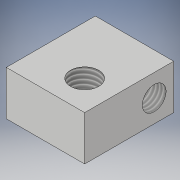
# Autodesk Inventor part: КВ33.000.109 - Каретка
Saved by Autodesk Inventor 2019 (Build 230136000, 136)
## iProperties
Created: 2021-04-04
Part Number: КВ33.000.109 - Каретка
Material: Типовые
Document SubType Name: Modeling
Designer: Петров Иван
Density: 1 g/cm^3
Appearance: По умолчанию
Mass: 10.7217 g
Surface Area: 35.9412 cm^2
Volume: 10.7217 cm^3
Author: Петров Иван
Autodesk Inventor part; units mm, degrees
ref_plane "YZ Plane" through (0, 0, 0) normal (1, 0, 0) x (0, 1, 0)
ref_plane "XZ Plane" through (0, 0, 0) normal (0, 1, 0) x (-1, 0, 0)
ref_plane "XY Plane" through (0, 0, 0) normal (0, 0, 1) x (1, 0, 0)
sketch "Sketch1" plane through (0, 0, 0) normal (0, 1, 0) x (-1, 0, 0)
  line L0 (0, 0) -> (26.4, 0)
  line L1 (26.4, 0) -> (26.4, -30)
  line L2 (26.4, -30) -> (0, -30)
  line L3 (0, -30) -> (0, 0)
  dimension "d0" = 26.4
  dimension "d1" = 30
  constraints: 8 end point, 2 parallel, 1 horizontal, 1 perpendicular
  measures "d0" distance of L1.end L2.end
  measures "d1" distance between parallel lines of L2 L0
extrude "Extrusion1" add sketch "Sketch1" along normal blind 15
sketch "Sketch2" plane through (0, 15, 0) normal (0, 1, 0) x (1, 0, 0)
  circle A0 centre (-10, 10) radius 4.75
  line L0 (0, 0) -> (0, 30) projected
  line L1 (-26.4, 0) -> (0, 0) projected
  dimension "d4" = 9.5
  dimension "d5" = 10
  dimension "d6" = 10
  constraints: 1 centre point
  measures "d4" diameter of A0
  measures "d5" distance from line of L0 A0.centre
  measures "d6" distance from line of L1 A0.centre
extrude "Extrusion2" cut sketch "Sketch2" against normal blind 15
sketch "Sketch3" plane through (-26.4, 0, -30) normal (-1, 0, 0) x (0, 0, 1)
  line L0 (24.75, 0) -> (15.25, 0) projected
  line L1 (15.25, 15) -> (24.75, 15) projected
  line L2 (24.75, 15) -> (24.75, 0) projected
  line L3 (15.25, 15) -> (15.25, 0) projected
  circle A0 centre (20, 7.5) radius 2
  point P0 (30, 0)
  dimension "d12" = 4
  constraints: 1 centre point
  measures "d12" diameter of A0
hole "Hole1" at (-26.4, 7.5, -10) direction (1, 0, 0) diameter 6 depth 8 tip angle 120
sketch "Sketch4" plane through (-26.4, 0, -30) normal (-1, 0, 0) x (0, 0, 1)
  line L0 (0, 0) -> (0, 15) projected
  circle A0 centre (6.5597, 7.5) radius 4
  point P0 (30, 0)
  dimension "d20" = 8
  constraints: 1 centre point
  measures "d20" diameter of A0
extrude "Extrusion3" cut sketch "Sketch4" against normal blind 32.75
thread "Thread1" size "M10x1.5" class "6H" standard "ANSI Metric M Profile" full length
thread "Thread2" size "M8x1.25" class "6H" standard "ANSI Metric M Profile" full length
body "Solid1"
